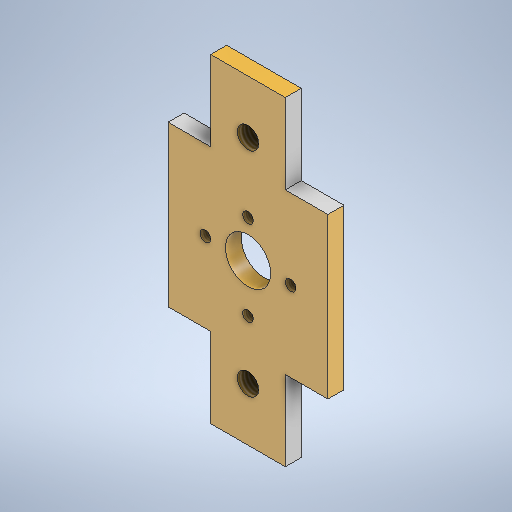
# Autodesk Inventor part: placa_soporte_motor
Saved by Autodesk Inventor 2026 (Build 300175050, 175E)
## iProperties
Created: 2025-08-22
Part Number: placa_soporte_motor
Material: Genérico
Document SubType Name: Modeling
Designer: piero
Density: 1 g/cm^3
Appearance: Valor por defecto
Author: piero
Autodesk Inventor part; units mm, degrees
ref_plane "YZ Plane" through (0, 0, 0) normal (1, 0, 0) x (0, 1, 0)
ref_plane "XZ Plane" through (0, 0, 0) normal (0, 1, 0) x (-1, 0, 0)
ref_plane "XY Plane" through (0, 0, 0) normal (0, 0, 1) x (1, 0, 0)
sketch "Boceto1" plane through (0, 0, 0) normal (0, 0, 1) x (1, 0, 0)
  line L0 (0, 0) -> (30, 0)
  line L1 (30, 0) -> (30, 60)
  line L2 (30, 60) -> (0, 60)
  line L3 (0, 60) -> (0, 0)
  circle A0 centre (15, 30) radius 4.25
  circle A1 centre (7, 30) radius 1
  circle A2 centre (23, 30) radius 1
  circle A3 centre (15, 37) radius 1
  circle A4 centre (15, 21) radius 1
  circle A5 centre (15, 50) radius 2
  circle A6 centre (15, 10) radius 2
  point P0 (15, 0)
  dimension "d0" = 30
  dimension "d1" = 60
  dimension "d2" = 8.5
  dimension "d3" = 2
  dimension "d4" = 2
  dimension "d7" = 2
  dimension "d8" = 2
  dimension "d9" = 16
  dimension "d21" = 30
  dimension "d22" = 23
  dimension "d24" = 0
  dimension "d25" = 0
  dimension "d26" = 16
  dimension "d27" = 7
  dimension "d28" = 4
  dimension "d29" = 4
  dimension "d30" = 20
  dimension "d31" = 20
  constraints: 8 end point, 7 centre point, 2 parallel, 1 horizontal, 1 midpoint, 1 perpendicular
  measures "d0" distance of L2.end L1.end
  measures "d1" distance of L1.end L0.end
  measures "d2" diameter of A0
  measures "d3" diameter of A1
  measures "d4" diameter of A2
  measures "d7" diameter of A3
  measures "d8" diameter of A4
  measures "d9" distance of A4.centre A3.centre
  measures "d21" distance from line of L2 A0.centre
  measures "d22" distance from line of L2 A3.centre
  measures "d24" vertical distance of A0.centre A1.centre
  measures "d25" vertical distance of A0.centre A2.centre
  measures "d26" distance of A2.centre A1.centre
  measures "d27" distance from line of L3 A1.centre
  measures "d28" diameter of A5
  measures "d29" diameter of A6
  measures "d30" distance of A5.centre A0.centre
  measures "d31" distance of A6.centre A0.centre
extrude "Extrusión1" add sketch "Boceto1" along normal blind 3
thread "Rosca1" size "M2x0.4" class "6H" standard "ANSI Metric M Profile" full length
thread "Rosca2" size "M2x0.4" class "6H" standard "ANSI Metric M Profile" full length
thread "Rosca3" size "M2x0.4" class "6H" standard "ANSI Metric M Profile" full length
thread "Rosca4" size "M2x0.4" class "6H" standard "ANSI Metric M Profile" full length
thread "Rosca5" size "M4x0.7" class "6H" standard "ANSI Metric M Profile" full length
thread "Rosca6" size "M4x0.7" class "6H" standard "ANSI Metric M Profile" full length
sketch "Boceto2" plane through (0, 0, 3) normal (0, 0, 1) x (1, 0, 0)
  line L0 (30, 60) -> (0, 60) projected
  line L1 (0, 60) -> (8, 60)
  line L2 (8, 60) -> (8, 45)
  line L3 (8, 45) -> (0, 45)
  line L4 (0, 45) -> (0, 60)
  line L5 (30, 60) -> (22, 60)
  line L6 (22, 60) -> (22, 45)
  line L7 (22, 45) -> (30, 45)
  line L8 (30, 45) -> (30, 60)
  line L9 (0, 0) -> (30, 0) projected
  line L10 (0, 0) -> (8, 0)
  line L11 (8, 0) -> (8, 15)
  line L12 (8, 15) -> (0, 15)
  line L13 (0, 15) -> (0, 0)
  line L14 (30, 0) -> (22, 0)
  line L15 (22, 0) -> (22, 15)
  line L16 (22, 15) -> (30, 15)
  line L17 (30, 15) -> (30, 0)
  dimension "d36" = 8
  dimension "d37" = 15
  dimension "d38" = 8
  dimension "d39" = 15
  dimension "d40" = 8
  dimension "d41" = 15
  dimension "d42" = 8
  dimension "d43" = 15
  constraints: 32 end point, 8 parallel, 4 horizontal, 4 perpendicular
  measures "d36" distance of L2.end L3.end
  measures "d37" distance of L1.end L2.end
  measures "d38" distance of L7.end L6.end
  measures "d39" distance of L6.end L5.end
  measures "d40" distance of L12.end L11.end
  measures "d41" distance of L11.end L10.end
  measures "d42" distance of L15.end L16.end
  measures "d43" distance of L14.end L15.end
extrude "Extrusión2" cut sketch "Boceto2" against normal blind 3
